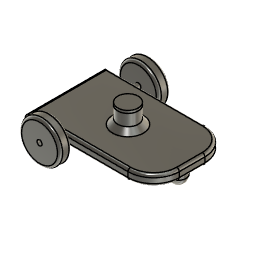
SimpleBot (Autodesk Fusion 360 design; units mm, degrees)
Autodesk Fusion 360 part; units mm, degrees
sketch "Sketch1" plane through (0, 0, 0) normal (0, 0, 1) x (1, 0, 0)
  line L0 (250, -150) -> (-250, -150)
  line L1 (-250, -150) -> (-250, 150)
  line L2 (-250, 150) -> (250, 150)
  line L3 (250, 150) -> (250, -150)
  line L4 (250, -150) -> (-250, 150) construction
  line L5 (-250, -150) -> (250, 150) construction
  dimension "d1" = 500
  dimension "d2" = 300
  constraint horizontal L0
  constraint perpendicular L0 L1
  constraint parallel L0 L2
  constraint parallel L1 L3
  constraint coincident L4 origin
  constraint coincident L5 origin
  measures "d1" distance of L1.end L2.end
  measures "d2" distance of L0.end L1.end
extrude "Extrude1" add sketch "Sketch1" along normal blind 40 makes body 1
sketch "Sketch2" plane through (0, -150, 0) normal (0, -1, 0) x (1, 0, 0)
  line L0 (-250, 0) -> (250, 0)
  line L1 (250, 0) -> (250, 40)
  line L2 (250, 40) -> (-250, 40)
  line L3 (-250, 40) -> (-250, 0)
  line L4 (-250, 20) -> (-130, 20) construction
  circle A0 centre (-130, 20) radius 10
  dimension "d5" = 120
  dimension "d6" = 20
  constraint midpoint L3 L4.start
  constraint perpendicular L3 L4
  constraint coincident L4.end A0.centre
  measures "d5" distance of L4.start L4.end
  measures "d6" diameter of A0
extrude "Extrude2" add sketch "Sketch2" along normal blind 20 contours A0 bodies 1
mirror "Mirror1" about plane through (0, 0, 0) normal (0, 1, 0) of "Extrude2"
sketch "Sketch3" plane through (0, -170, 0) normal (0, -1, 0) x (1, 0, 0)
  circle A0 centre (-130, 20) radius 10
  circle A1 centre (-130, 20) radius 80
  dimension "d11" = 160
  constraint concentric A0 A1
  measures "d11" diameter of A1
extrude "Extrude3" add sketch "Sketch3" along normal blind 45 separate body makes body 2
mirror "Mirror2" about plane through (0, 0, 0) normal (0, 1, 0) of "Extrude3" makes body 3
ref_plane "WorkPlane1" through (-130, -186.385, -60) normal (0, 0, -1) x (-1, 0, 0)
move_body "Move1" bodies 1 2 3 to x (1, 0, 0) y (0, 1, 0) z (0, 0, 1) at (0, 0, 60)
sketch "Sketch4" plane through (0, 0, 60) normal (0, 0, -1) x (1, 0, 0)
  line L0 (-250, -150) -> (250, -150)
  line L1 (250, -150) -> (250, 150)
  line L2 (250, 150) -> (-250, 150)
  line L3 (-250, 150) -> (-250, -150)
  line L4 (250, 0) -> (200, 0)
  circle A0 centre (200, 0) radius 30
  dimension "d17" = 50
  dimension "d18" = 60
  constraint midpoint L1 L4.start
  constraint perpendicular L1 L4
  constraint coincident L4.end A0.centre
  measures "d17" distance of L4.start L4.end
  measures "d18" diameter of A0
extrude "Extrude4" add sketch "Sketch4" along normal blind 60 separate body contours A0 makes body 4
fillet "Fillet1" radius 30 1 faces at (190.9903, -4.3388, 0) on bodies 4
fillet "Fillet2" radius 10 1 edges at (172.0302, 10.8485, 60) on bodies 4
fillet "Fillet3" radius 100 2 edges at (250, -150, 80) (250, 150, 80) on bodies 1
chamfer "Chamfer1" distance 20 angle 45 1 edges at (-250, 0, 100) on bodies 1
sketch "Sketch5" plane through (0, 0, 100) normal (0, 0, 1) x (-1, 0, 0)
  line L0 (230, -150) -> (230, 150)
  line L1 (230, 150) -> (-150, 150)
  arc A0 (-150, 150) -> (-250, 50) centre (-150, 50) ccw
  line L2 (-250, 50) -> (-250, -50)
  arc A1 (-250, -50) -> (-150, -150) centre (-150, -50) ccw
  line L3 (-150, -150) -> (230, -150)
  circle A2 centre (0, 0) radius 40
  dimension "d28" = 80
  constraint coincident A2.centre origin
  measures "d28" diameter of A2
extrude "Extrude5" add sketch "Sketch5" along normal blind 65 contours A2 bodies 1
sketch "Sketch8" plane through (0, 0, 165) normal (0, 0, 1) x (-1, 0, 0)
  circle A0 centre (0, 0) radius 40
  circle A1 centre (0, 0) radius 40
  constraint coincident A0.centre A1.centre
extrude "Extrude6" add sketch "Sketch8" along normal blind 10 separate body makes body 5
fillet "Fillet4" radius 10 17 edges at (-40, -150, 100) (220.7107, -120.7107, 100) (250, 0, 100) (220.7107, 120.7107, 100) (-40, 150, 100) (-50, -150, 60) (220.7107, -120.7107, 60) (250, 0, 60) (220.7107, 120.7107, 60) (-50, 150, 60) (-230, 0, 100) (-250, 0, 80) (-250, 0, 60) (-204.5862, -215, 51.0708) (-204.5862, -170, 51.0708) (-204.5862, 170, 51.0708) (-204.5862, 215, 51.0708) on bodies 1 2 3
chamfer "Chamfer2" distance 20 angle 45 1 edges at (37.2931, -14.4646, 100) on bodies 1
copy_body "Body->Comp1" bodies 1 removing the originals makes body 6 in component "old_component"
copy_body "Body->Comp2" bodies 2 removing the originals makes body 7 in component "old_component (1)"
copy_body "Body->Comp3" bodies 3 removing the originals makes body 8 in component "old_component (2)"
copy_body "Body->Comp4" bodies 4 removing the originals makes body 9 in component "old_component (3)"
copy_body "Body->Comp5" bodies 5 removing the originals makes body 10 in component "old_component (4)"
copy_body "CopyPasteBodies1" bodies 6 makes body 11 in component "base_link"
copy_body "CopyPasteBodies1'" bodies 7 makes body 12 in component "right_wheel_1"
copy_body "CopyPasteBodies1''" bodies 8 makes body 13 in component "left_wheel_1"
copy_body "CopyPasteBodies1'''" bodies 9 body 9 seen with x (1, 0, 0) y (0, 1, 0) z (0, 0, 1) at (-4, 0, 0) makes body 14 in component "caster_wheel_1"
copy_body "CopyPasteBodies1''''" bodies 10 makes body 15 in component "lidar_1"
component "old_component" placed x (1, 0, 0) y (0, 1, 0) z (0, 0, 1) at (0, 0, 0)
component "old_component (1)" placed x (1, 0, 0) y (0, 1, 0) z (0, 0, 1) at (0, 0, 0)
component "old_component (2)" placed x (1, 0, 0) y (0, 1, 0) z (0, 0, 1) at (0, 0, 0)
component "old_component (3)" placed x (1, 0, 0) y (0, 1, 0) z (0, 0, 1) at (-4, 0, 0)
component "old_component (4)" placed x (1, 0, 0) y (0, 1, 0) z (0, 0, 1) at (0, 0, 0)
component "base_link" placed x (1, 0, 0) y (0, 1, 0) z (0, 0, 1) at (0, 0, 0)
component "right_wheel_1" placed x (1, 0, 0) y (0, 1, 0) z (0, 0, 1) at (0, 0, 0)
component "left_wheel_1" placed x (1, 0, 0) y (0, 1, 0) z (0, 0, 1) at (0, 0, 0)
component "caster_wheel_1" placed x (1, 0, 0) y (0, 1, 0) z (0, 0, 1) at (0, 0, 0)
component "lidar_1" placed x (1, 0, 0) y (0, 1, 0) z (0, 0, 1) at (0, 0, 0)
named bodies: "base_link", "right_wheel", "left_wheel", "caster_wheel", "lidar"
